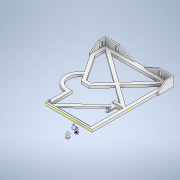
# Autodesk Inventor part: OscarNoring240sSkalV.1Microdator
Saved by Autodesk Inventor 2021 (Build 250183000, 183)
## iProperties
Created: 2024-10-09
Part Number: OscarNoring240sSkalV.1Microdator
Material: PBT Plastic
Document SubType Name: Modeling
Designer: 24oscnor
Density: 1.31 g/cm^3
Appearance: Smooth - White
Author: 24oscnor
Autodesk Inventor part; units mm, degrees
ref_plane "YZ Plane" through (0, 0, 0) normal (1, 0, 0) x (0, 1, 0)
ref_plane "XZ Plane" through (0, 0, 0) normal (0, 1, 0) x (-1, 0, 0)
ref_plane "XY Plane" through (0, 0, 0) normal (0, 0, 1) x (1, 0, 0)
sketch "Sketch1" plane through (0, 0, 0) normal (0, 1, 0) x (-1, 0, 0)
  line L0 (82, -54) -> (0, -54)
  line L1 (0, -54) -> (0, 0)
  line L2 (58, 44) -> (0, 44)
  line L3 (0, 44) -> (0, 0)
  circle A0 centre (56, 41) radius 1.45
  circle A1 centre (12.5, 13) radius 1.45
  line L4 (82, -54) -> (82, -35.896)
  line L5 (54.6748, -2.2232) -> (78, -37.11)
  line L6 (78, -37.11) -> (78, -50)
  line L7 (78, -50) -> (4, -50)
  line L8 (4, -50) -> (4, 0)
  line L9 (54, 40) -> (4, 40)
  line L10 (4, 40) -> (4, 0)
  line L11 (54.6748, -2.2232) -> (54, -1.214)
  line L12 (54, -1.214) -> (9.4186, -50)
  line L13 (4, -50) -> (48.5814, -1.214)
  line L14 (78, -50) -> (10.8081, -1.214)
  line L15 (4, -1.214) -> (71.1919, -50)
  line L16 (11.05, 13) -> (11.05, 9.6245)
  line L17 (13.95, 13) -> (13.95, 12.0261)
  line L18 (11.05, 9.6245) -> (11.05, 3.786)
  line L19 (13.95, 12.0261) -> (13.95, 3.786)
  line L20 (54, 40) -> (17.1403, 3.786)
  line L21 (13.95, 6.2591) -> (48.2925, 40)
  line L22 (3.6116, 3.786) -> (17.1403, 3.786)
  line L23 (4, -1.214) -> (17.1403, -1.214)
  line L24 (17.1403, -1.214) -> (17.1403, 3.786)
  line L25 (48.5814, -1.214) -> (54, -1.214)
  line L26 (44.9262, -5.214) -> (56.6744, -5.214)
  line L27 (58, 44) -> (58, 15)
  line L28 (58, 15) -> (54, 15)
  line L29 (54, 40) -> (54, 15)
  line L30 (54, -1.214) -> (58.8117, -1.214)
  line L31 (58.8117, -1.214) -> (82, -35.896)
  arc A2 (64.4344, -9.6237) -> (58, 15) centre (58, 1.8475) ccw
  arc A3 (67.2169, -12.6183) -> (58, 19) centre (58, 1.8475) ccw
  line L32 (67.2169, -12.6183) -> (66.6776, -12.9789)
  point P0 (4, 0)
  point P1 (4, 2.786)
  point P2 (54, 2.786)
  point P3 (10.2713, 40)
  point P4 (10.2713, 2.786)
  point P5 (47.7287, 40)
  point P6 (33.5153, -17.701)
  point P7 (30.7999, -20.6726)
  point P8 (34.0572, -23.0376)
  point P9 (36.7727, -20.0661)
  point P10 (13.95, 40)
  point P11 (19.4764, 40)
  point P12 (4, 3.786)
  point P13 (11.05, 3.786)
  point P14 (10.8081, -1.214)
  point P15 (50.3447, -5.214)
  point P16 (67.0734, -13.5707)
  dimension "d0" = 82
  dimension "d1" = 54
  dimension "d2" = 44
  dimension "d5" = 3
  dimension "d6" = 2.9
  dimension "d8" = 12.5
  dimension "d9" = 2.9
  dimension "d36" = 18.104
  dimension "d94" = 90
  dimension "d95" = 90
  dimension "d96" = 31
  dimension "d97" = 4
  dimension "d98" = 4
  dimension "d103" = 4
  dimension "d104" = 4
  dimension "d112" = 4
  dimension "d113" = 44.494
  dimension "d121" = 134.494
  dimension "d122" = 135.506
  dimension "d123" = 13.5287
  dimension "d124" = 13.1403
  dimension "d125" = 90
  dimension "d126" = 54.018
  dimension "d127" = 42.422
  dimension "d128" = 4
  dimension "d129" = 4
  dimension "d130" = 146.233
  dimension "d131" = 11.7482
  dimension "d132" = 25
  dimension "d133" = 51.673
  dimension "d134" = 4
  dimension "d140" = 2
  dimension "d141" = 17.1526
  dimension "d155" = 58
  constraints: 66 end point, 16 point on line, 7 point on circle, 6 parallel, 4 centre point, 4 perpendicular, 3 horizontal, 3 tangent, 3 vertical, 3 other
  measures "d0" distance of L0.start L0.end
  measures "d1" distance of L0.end L1.end
  measures "d2" distance of L2.end L1.end
  measures "d5" distance from line of L2 A0.centre
  measures "d6" diameter of A0
  measures "d8" distance from line of L3 A1.centre
  measures "d9" diameter of A1
  measures "d36" distance of L0.start L4.end
  measures "d94" angle of L1 L0
  measures "d95" angle of L4 L0
  measures "d96" distance from line of L2 A1.centre
  measures "d97" distance between parallel lines of L0 L7
  measures "d98" distance between parallel lines of L3 L10
  measures "d103" distance between parallel lines of L13 L12
  measures "d104" distance between parallel lines of L15 L14
  measures "d112" distance between parallel lines of L20 L21
  measures "d113" angle of L21 L9
  measures "d121" angle of L19 L21
  measures "d122" angle of L22 L20
  measures "d123" distance of L22.start L20.end
  measures "d124" distance of L15.start L23.end
  measures "d125" angle of L22 L10
  measures "d126" angle of L8 L15
  measures "d127" angle of L8 L13
  measures "d128" distance between parallel lines of L25 L26
  measures "d129" distance between parallel lines of L31 L5
  measures "d130" angle of L6 L5
  measures "d131" distance of L26.start L26.end
  measures "d132" distance of L9.start L28.end
  measures "d133" distance of L9.start L20.end
  measures "d134" radial gap between concentric circles of A3 A2
  measures "d140" distance from line of L27 A0.centre
  measures "d141" radius of A3
  measures "d155" distance of L2.start L2.end
extrude "Extrusion1" add sketch "Sketch1" along normal blind 1.5 contours L0 L1 L3 L2 L27 L28 L29 L9 L10 L8 L7 L6 L5 L11 L30 L31 L4 | L31 A2 L27 A3 L32 | L11 L5 L26 L12 | L12 L26 L13 L25 | L12 L14 L13 L26 | L20 L22 L19 L21 L9 | L14 L7 L15 L12 | L12 L15 L13 L14 | L24 L23 L8 L10 L22 | L12 L7 L13 L15 | L13 L15 L23 L14 | L19 L22 L18 L16 A1 L17 | A0
sketch "Sketch2" plane through (0, 0, -54) normal (0, 0, -1) x (-1, 0, 0)
  line L0 (58, 0) -> (0, 0) projected
  line L1 (0, 0) -> (82, 0)
  line L2 (0, 10) -> (0, 0)
  line L3 (12.24, 7.7) -> (16.44, 7.7)
  line L4 (16.44, 7.7) -> (16.44, 2.5)
  line L5 (16.44, 2.5) -> (12.24, 2.5)
  line L6 (12.24, 2.5) -> (12.24, 7.7)
  line L7 (0, 1.5) -> (82, 1.5) projected
  line L8 (41, 10) -> (41, 0) construction
  line L9 (0, 10) -> (16.44, 10)
  line L10 (16.44, 10) -> (34.5439, 1.5)
  line L11 (58, 1.5) -> (0, 1.5) projected
  line L12 (24, 0) -> (82, 0)
  line L13 (82, 0) -> (0, 0)
  line L14 (82, 10) -> (82, 0)
  line L15 (69.76, 7.7) -> (65.56, 7.7)
  line L16 (65.56, 7.7) -> (65.56, 2.5)
  line L17 (65.56, 2.5) -> (69.76, 2.5)
  line L18 (69.76, 2.5) -> (69.76, 7.7)
  line L19 (82, 1.5) -> (0, 1.5)
  line L20 (82, 10) -> (65.56, 10)
  line L21 (65.56, 10) -> (47.4561, 1.5)
  line L22 (24, 1.5) -> (82, 1.5)
  line L23 (0, 0) -> (0, 1.5) projected
  line L24 (0, 0) -> (82, 0)
  line L25 (82, 0) -> (82, -1.5)
  line L26 (82, -1.5) -> (0, -1.5)
  line L27 (0, -1.5) -> (0, 0)
  point P0 (47.4561, 1.5)
  dimension "d13" = 10
  dimension "d14" = 12.24
  dimension "d16" = 4.2
  dimension "d17" = 5.2
  dimension "d18" = 1
  dimension "d34" = 20
  dimension "d35" = 16.44
  dimension "d137" = 1.5
  constraints: 48 end point, 13 symmetric about line, 4 horizontal, 4 parallel, 2 perpendicular, 2 point on line, 1 midpoint
  measures "d13" distance of L2.start L0.end
  measures "d14" distance between parallel lines of L2 L6
  measures "d16" distance of L4.end L5.end
  measures "d17" distance of L5.end L3.start
  measures "d18" distance between parallel lines of L5 L7
  measures "d34" distance of L9.end L10.end
  measures "d35" distance of L2.start L9.end
  measures "d137" distance of L24.end L25.end
extrude "Extrusion2" add sketch "Sketch2" along normal blind 1.5
sketch "Sketch4" plane through (0, 1.5, -54) normal (1, 0, 0) x (0, 0, -1)
  line L0 (0, 0) -> (0, 8.5) projected
  line L1 (-98, 0) -> (0, 0) projected
  line L2 (-18.104, 0) -> (-18.104, -1.5)
  line L3 (-98, -1.5) -> (0, -1.5) projected
  line L4 (0, 8.5) -> (1.5, 8.5) projected
  line L5 (0, 8.5) -> (-7.2, 8.5)
  line L6 (0, 0) -> (-18.104, 0) projected
  line L7 (-7.2, 8.5) -> (-18.104, 0)
  line L8 (0, -1.5) -> (-18.104, -1.5) projected
  line L9 (-18.104, -1.5) -> (1.5, -1.5)
  line L10 (0, 0) -> (1.5, 0) projected
  line L11 (1.5, -1.5) -> (1.5, 0)
  line L12 (1.5, 0) -> (-18.104, 0)
  line L13 (1.5, 0) -> (1.5, 8.5)
  line L14 (0, 8.5) -> (1.5, 8.5) projected
  line L15 (1.5, 8.5) -> (0, 8.5)
  line L16 (-18.104, -1.5) -> (-18.104, 0) projected
  line L17 (-18.104, -1.5) -> (-18.104, -3)
  line L18 (-18.104, -3) -> (1.5, -3)
  line L19 (1.5, -3) -> (1.5, -1.5)
  point P0 (-54, -1.5)
  dimension "d135" = 7.2
  dimension "d136" = 1.5
  constraints: 22 end point, 4 perpendicular, 3 point on line, 2 collinear, 2 horizontal, 1 parallel, 1 vertical
  measures "d135" distance of L0.end L5.end
  measures "d136" distance between parallel lines of L3 L18
extrude "Extrusion3" add sketch "Sketch4" along normal blind 1.5 contours L1 L7 L5 L0 | L0 L4 L13 L10 | L3 L9 L19 L18 L17
sketch "Sketch6" plane through (0, 0, -55.5) normal (1, 0, 0) x (0, 0, -1)
  line L0 (-99.5, 1.5) -> (-19.604, 1.5) projected
  line L1 (-19.6039, 1.5) -> (-19.6039, 0)
  line L2 (-99.5, 0) -> (-19.604, 0) projected
  line L3 (-19.6039, 0) -> (0, 0)
  line L4 (-1.5, 10) -> (0, 10) projected
  line L5 (0, 0) -> (0, 10)
  line L6 (-19.6039, 1.5) -> (-1.5, 1.5)
  line L7 (-1.5, 1.5) -> (-1.5, 10) projected
  line L8 (-1.5, 10) -> (-1.5, 1.5)
  line L9 (0, 10) -> (-1.5, 10)
  point P0 (-55.5, 0)
  point P1 (-1.5, 0)
  point P2 (-1.5, 0)
  constraints: 12 end point, 2 collinear, 1 horizontal, 1 perpendicular, 1 point on line, 1 vertical
extrude "Extrusion4" add sketch "Sketch6" along normal blind 1.5
sketch "Sketch7" plane through (-82, 0, 0) normal (-1, 0, 0) x (0, 0, 1)
  line L0 (-54, 10) -> (-35.8961, 1.5)
  line L1 (-35.8961, 1.5) -> (-35.8961, 0)
  line L2 (0, 0) -> (-55.5, 0) projected
  line L3 (-35.8961, 0) -> (-55.5, 0)
  line L4 (-55.5, 0) -> (-55.5, 10)
  line L5 (-55.5, 10) -> (-54, 10)
  line L6 (-51, 8) -> (-46.5, 8)
  line L7 (-46.5, 8) -> (-46.5, 2.5)
  line L8 (-46.5, 2.5) -> (-51, 2.5)
  line L9 (-51, 2.5) -> (-51, 8)
  line L10 (-54, 1.5) -> (0, 1.5) projected
  line L11 (-54, 10) -> (-46.8, 10)
  line L12 (-35.896, 1.5) -> (-35.8961, 1.5) projected
  line L13 (-46.8, 10) -> (-35.8961, 1.5)
  line L14 (-55.5, 0) -> (-35.896, 0)
  line L15 (-35.896, 0) -> (-35.896, -1.5)
  line L16 (-35.896, -1.5) -> (-55.5, -1.5)
  line L17 (-55.5, -1.5) -> (-55.5, 0)
  point P0 (-54, 0)
  point P1 (-54, 0)
  dimension "d26" = 4.5
  dimension "d27" = 4.5
  dimension "d28" = 5.5
  dimension "d29" = 1
  dimension "d30" = 13.8255
  constraints: 30 end point, 4 parallel, 4 perpendicular, 3 horizontal, 1 point on line, 1 vertical
  measures "d26" distance between parallel lines of L4 L9
  measures "d27" distance between parallel lines of L9 L7
  measures "d28" distance of L8.end L6.start
  measures "d29" distance between parallel lines of L8 L10
  measures "d30" distance of L11.end L0.end
extrude "Extrusion5" add sketch "Sketch7" along normal blind 1.5 contours L11 L13 L0 L7 L6 | L0 L6 L9 L8 L7 L1 L2 L4 L5 | L2 L15 L16 L17
extrude "Extrusion6" add sketch "Sketch1" along normal blind 3 contours A1 | A0
sketch "Sketch15" plane through (-56, 3, 41) normal (0, 1, 0) x (1, 0, 0)
  circle A0 centre (0, 0) radius 1.45 projected
  circle A1 centre (0, 0) radius 0.85
  arc A2 (42.05, 28) -> (44.95, 28) centre (43.5, 28) ccw projected
  circle A3 centre (43.5, 28) radius 0.9
  point P0 (56, 41)
  dimension "d76" = 1.7
  dimension "d110" = 1.8
  constraints: 2 centre point, 2 coincident
  measures "d76" diameter of A1
  measures "d110" diameter of A3
extrude "Extrusion10" cut sketch "Sketch15" against normal up to surface (3 mm away) contours A1 | A3
sketch "Sketch16" plane through (0, 0, 0) normal (0, 1, 0) x (-1, 0, 0)
  circle A0 centre (9.3309, 54.4237) radius 2
  circle A1 centre (9.3309, 54.4237) radius 0.65
  line L0 (58, 44) -> (0, 44) projected
  line L1 (7.831, 59.7931) -> (15.9352, 59.7931) construction
  circle A2 centre (9.3309, 65.1624) radius 2
  circle A3 centre (9.3309, 65.1624) radius 0.65
  point P0 (0, 0)
  dimension "d80" = 4
  dimension "d81" = 1.3
  constraints: 4 centre point, 2 coincident, 2 end point, 2 symmetric about line, 1 horizontal, 2 other
  measures "d80" diameter of A0
  measures "d81" diameter of A1
extrude "Extrusion11" add sketch "Sketch16" along normal blind 2 contours A2 | A3
extrude "Extrusion12" add sketch "Sketch16" along normal blind 2 contours A0 | A1
extrude "Extrusion13" add sketch "Sketch16" along normal blind 5 contours A1 | A3
extrude "Extrusion14" add sketch "Sketch1" against normal blind 1.5 contours L31 A2 L27 A3 L32 | L11 L5 L26 L12 | L12 L26 L13 L25 | L12 L14 L13 L26 | L20 L22 L19 L21 L9 | L14 L7 L15 L12 | L12 L15 L13 L14 | L24 L23 L8 L10 L22 | L12 L7 L13 L15 | L13 L15 L23 L14 | L19 L22 L18 L16 A1 L17
extrude "Extrusion15" [suppressed]
extrude "Extrusion16" add sketch "Sketch1" against normal blind 1.5 contours L0 L1 L3 L2 L27 L28 L29 L9 L10 L8 L7 L6 L5 L11 L30 L31 L4 | L12 L26 L13 L25 | L12 L14 L13 L26 | L20 L22 L19 L21 L9 | L12 L15 L13 L14 | L24 L23 L8 L10 L22 | L12 L7 L13 L15 | L13 L15 L23 L14 | L19 L22 L18 L16 A1 L17
sketch "Sketch24" plane through (0, 0, 0) normal (0, -1, 0) x (1, 0, 0)
  point P0 (0, 0)
extrude "Extrusion17" add sketch "Sketch16" against normal blind 1.5 contours A0 | A1 | A2 | A3
sketch "Sketch25" plane through (0, 1.5, 0) normal (0, 1, 0) x (1, 0, 0)
  line L0 (-4, -3.786) -> (-4, -40) projected
  line L1 (-4, -3.786) -> (-4, -1.786)
  line L2 (-4, -1.786) -> (-7.525, -1.786)
  line L3 (-11.05, -3.786) -> (-4, -3.786) projected
  line L4 (-7.525, -1.786) -> (-17.1403, -1.786)
  line L5 (-17.1403, -3.786) -> (-17.1403, 1.214) projected
  line L6 (-17.1403, -1.786) -> (-17.1403, -3.786)
  line L7 (-17.1403, -3.786) -> (-51.0593, -37.1109)
  line L8 (-54, -40) -> (-17.1403, -3.786) projected
  line L9 (-48.2925, -40) -> (-13.95, -6.2591) projected
  line L10 (-48.256, -39.9642) -> (-13.95, -6.2591)
  line L11 (-13.95, -6.2591) -> (-13.95, -10.786)
  line L12 (-13.95, -6.2591) -> (-13.95, -13) projected
  line L13 (-13.95, -10.786) -> (-11.05, -10.786)
  line L14 (-11.05, -13) -> (-11.05, -3.786) projected
  line L15 (-11.05, -10.786) -> (-11.05, -3.786)
  line L16 (-11.05, -3.786) -> (-7.525, -3.786)
  line L17 (-4, -3.786) -> (-7.525, -3.786)
  line L18 (-51.0593, -37.1109) -> (-54, -40)
  line L19 (-54, -15) -> (-54, -40) projected
  line L20 (-48.2925, -40) -> (-54, -40)
  point P0 (0, 0)
  dimension "d142" = 2
  dimension "d143" = 45.506
  dimension "d144" = 7
  constraints: 26 end point, 5 point on line, 4 perpendicular, 2 collinear, 2 horizontal, 2 vertical, 1 midpoint
  measures "d142" distance of L16.end L2.end
  measures "d143" angle of L12 L10
  measures "d144" distance of L3.start L13.end
extrude "Extrusion18" cut sketch "Sketch25" against normal blind 1.5
sketch "Sketch26" plane through (0, 0, 0) normal (0, -1, 0) x (1, 0, 0)
  arc A0 (-11.05, 13) -> (-13.95, 13) centre (-12.5, 13) ccw projected
  circle A1 centre (-12.5, 13) radius 1.45
  circle A2 centre (-12.5, 13) radius 0.85
  point P0 (0, 0)
  constraints: 2 coincident, 1 centre point, 3 other
extrude "Extrusion19" add sketch "Sketch26" along normal blind 1.5
sketch "Sketch27" plane through (0, 1.5, 0) normal (0, 1, 0) x (1, 0, 0)
  line L0 (-48.2925, -40) -> (-4, -40) projected
  line L1 (-4, -40) -> (-54.05, -40)
  line L2 (-54.05, -40) -> (-54.05, -42)
  line L3 (-54.05, -42) -> (-4, -42)
  line L4 (-4, -42) -> (-4, -40)
  line L5 (-54, -40) -> (-54, -15) projected
  circle A0 centre (-56, -41) radius 1.45 projected
  point P0 (0, 0)
  dimension "d150" = 2
  dimension "d154" = 0.5
  constraints: 8 end point, 2 parallel, 1 horizontal, 1 perpendicular
  measures "d150" distance between parallel lines of L0 L3
  measures "d154" distance edge to line of A0 L2
extrude "Extrusion20" cut sketch "Sketch27" against normal blind 1.5 contours L0 L4 L3 L2 L1
body "Solid1"
